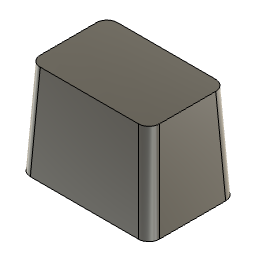
BUTTON_FINAL v1 (Autodesk Fusion 360 design; units mm, degrees)
Autodesk Fusion 360 part; units mm, degrees
sketch "Sketch1" plane through (0, 0, 0) normal (0, 0, 1) x (1, 0, 0) in component "BASE"
  line L0 (-50, 28.33) -> (-37.66, 28.33)
  line L1 (-37.66, 28.33) -> (-37.66, 20)
  line L2 (-37.66, 20) -> (-50, 20)
  line L3 (-50, 20) -> (-50, 28.33)
  dimension "d1" = 12.34
  dimension "d2" = 8.33
  constraint horizontal L0
  constraint perpendicular L0 L1
  constraint perpendicular L1 L2
  constraint perpendicular L0 L3
  measures "d1" distance of L0.start L0.end
  measures "d2" distance of L0.end L1.end
extrude "Extrude1" add sketch "Sketch1" along normal blind 9.07 draft -3 in component "BASE"
fillet "Fillet1" radius 1 1 edges at (-37.8977, 28.0923, 4.535) in component "BASE"
fillet "Fillet2" radius 1 1 edges at (-37.8977, 20.2377, 4.535) in component "BASE"
fillet "Fillet3" radius 1 1 edges at (-49.7623, 28.0923, 4.535) in component "BASE"
fillet "Fillet4" radius 1 1 edges at (-49.7623, 20.2377, 4.535) in component "BASE"
sketch "Sketch2" plane through (0, 0, 0) normal (0, 0, -1) x (1, 0, 0) in component "BASE"
  ellipse E0 centre (-48.9986, -21.0014) end of major axis (-49.7077, -20.2923) minor radius 1 (-49.0014, -20) -> (-50, -20.9986) ccw
  line L0 (-50, -20.9986) -> (-50, -27.3314)
  ellipse E1 centre (-48.9986, -27.3286) end of major axis (-49.7077, -28.0377) minor radius 1 (-50, -27.3314) -> (-49.0014, -28.33) ccw
  line L1 (-49.0014, -28.33) -> (-38.6586, -28.33)
  ellipse E2 centre (-38.6614, -27.3286) end of major axis (-37.9523, -28.0377) minor radius 1 (-38.6586, -28.33) -> (-37.66, -27.3314) ccw
  line L2 (-37.66, -27.3314) -> (-37.66, -20.9986)
  ellipse E3 centre (-38.6614, -21.0014) end of major axis (-37.9523, -20.2923) minor radius 1 (-37.66, -20.9986) -> (-38.6586, -20) ccw
  line L3 (-38.6586, -20) -> (-49.0014, -20)
  line L4 (-48.9617, -22.2599) -> (-48.0617, -22.2599)
  line L5 (-48.0617, -22.2599) -> (-48.0617, -26.2729)
  line L6 (-48.0617, -26.2729) -> (-48.9617, -26.2729)
  line L7 (-48.9617, -26.2729) -> (-48.9617, -22.2599)
  line L8 (-39.4673, -22.3108) -> (-38.5673, -22.3108)
  line L9 (-38.5673, -22.3108) -> (-38.5673, -26.3238)
  line L10 (-38.5673, -26.3238) -> (-39.4673, -26.3238)
  line L11 (-39.4673, -26.3238) -> (-39.4673, -22.3108)
  dimension "d17" = 0.9
  dimension "d18" = 0.9
  dimension "d37" = 4.013
  dimension "d38" = 4.013
  constraint horizontal L4
  constraint vertical L5
  constraint horizontal L6
  constraint vertical L7
  constraint horizontal L8
  constraint vertical L9
  constraint horizontal L10
  constraint vertical L11
  measures "d17" distance of L4.start L4.end
  measures "d18" distance of L8.start L8.end
  measures "d37" distance of L8.start L10.end
  measures "d38" distance of L4.end L5.end
sketch "Sketch3" plane through (0, 0, 0) normal (0, 0, -1) x (1, 0, 0) in component "BASE"
  line L0 (-43.1934, -21.12) -> (-44.4133, -21.12)
  line L1 (-44.4133, -21.12) -> (-44.4133, -22.3399)
  line L2 (-44.4133, -22.3399) -> (-45.6332, -22.3399)
  line L3 (-45.6332, -22.3399) -> (-45.6332, -23.5598)
  line L4 (-45.6332, -23.5598) -> (-46.8531, -23.5598)
  line L5 (-46.8531, -23.5598) -> (-46.8531, -24.7797)
  line L6 (-46.8531, -24.7797) -> (-45.6332, -24.7797)
  line L7 (-45.6332, -24.7797) -> (-45.6332, -25.9996)
  line L8 (-45.6332, -25.9996) -> (-44.4133, -25.9996)
  line L9 (-44.4133, -25.9996) -> (-44.4133, -27.2195)
  line L10 (-44.4133, -27.2195) -> (-43.1934, -27.2195)
  line L11 (-43.1934, -27.2195) -> (-43.1934, -26.0138)
  line L12 (-43.1934, -26.0138) -> (-41.9735, -26.0138)
  line L13 (-41.9735, -26.0138) -> (-41.9735, -24.7939)
  line L14 (-41.9735, -24.7939) -> (-40.7536, -24.7939)
  line L15 (-40.7536, -24.7939) -> (-40.7536, -23.574)
  line L16 (-40.7536, -23.574) -> (-41.9735, -23.574)
  line L17 (-41.9735, -23.574) -> (-41.9735, -22.3541)
  line L18 (-41.9735, -22.3541) -> (-43.1934, -22.3541)
  line L19 (-43.1934, -22.3541) -> (-43.1934, -21.12)
  point P0 (-43.8034, -24.184)
  constraint perpendicular L0 L1
  constraint perpendicular L3 L4
  constraint perpendicular L4 L5
  constraint perpendicular L5 L6
  constraint perpendicular L6 L7
  constraint perpendicular L7 L8
  constraint perpendicular L8 L9
  constraint perpendicular L9 L10
  constraint perpendicular L8 L11
  constraint perpendicular L11 L12
  constraint perpendicular L12 L13
  constraint perpendicular L13 L14
  constraint perpendicular L14 L15
  constraint perpendicular L15 L16
  constraint perpendicular L16 L17
  constraint perpendicular L17 L18
extrude "Extrude2" cut sketch "Sketch2" sketch "Sketch3" along normal blind 0 and the other way blind 8.57 contours L4 L5 L6 L7 | L8 L9 L10 L11 of sketch 2 in component "BASE"
move_face "MoveFace1" by (0.0343, 1.0407, 0) 1 faces at (-44.4133, 24.3778, 8.57) in component "BASE"
sketch "Sketch4" plane through (0, 19.9452, -1.0453) normal (0, -0.99863, 0.052336) x (1, 0, 0) in component "BASE"
  line L0 (-48.526, 10.1292) -> (-49.0014, 1.0467)
  line L1 (-49.0014, 1.0467) -> (-38.6586, 1.0467)
  line L2 (-38.6586, 1.0467) -> (-39.134, 10.1292)
  line L3 (-39.134, 10.1292) -> (-48.526, 10.1292)
  line L4 (-40.5, 7.5) -> (-47.5, 7.5) construction
  line L5 (-47.5, 7.5) -> (-47.5, 2.5) construction
  line L6 (-47.5, 2.5) -> (-40.5, 2.5) construction
  line L7 (-40.5, 2.5) -> (-40.5, 7.5) construction
  dimension "d43" = 1
component "BASE" placed x (1, 0, 0) y (0, 1, 0) z (0, 0, 1) at (0, 0, 0)
